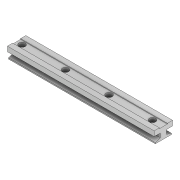
# Autodesk Inventor part: Rail
Saved by Autodesk Inventor 2020 (Build 240168000, 168)
## iProperties
Created: 2020-10-06
Part Number: Rail
Material: Generic
Document SubType Name: Modeling
Designer: ferrerx
Density: 1 g/cm^3
Appearance: Aluminum - Polished
Mass: 26.2987 g
Surface Area: 169.014 cm^2
Volume: 26.2987 cm^3
Author: ferrerx
Autodesk Inventor part; units mm, degrees
ref_plane "YZ Plane" through (0, 0, 0) normal (1, 0, 0) x (0, 1, 0)
ref_plane "XZ Plane" through (0, 0, 0) normal (0, 1, 0) x (-1, 0, 0)
ref_plane "XY Plane" through (0, 0, 0) normal (0, 0, 1) x (1, 0, 0)
sketch "Sketch1" plane through (0, 0, 0) normal (1, 0, 0) x (0, 1, 0)
  line L0 (0, 0) -> (0, -7.42)
  line L1 (0, -7.42) -> (1.0563, -7.42)
  line L2 (1.0563, -7.42) -> (2.51, -2.84)
  line L3 (2.51, -2.84) -> (6.31, -2.84)
  line L4 (6.31, -2.84) -> (6.31, -8.45)
  line L5 (6.31, -8.45) -> (10.81, -8.45)
  line L6 (10.81, -8.45) -> (10.81, -3.65)
  line L7 (10.81, -3.65) -> (10.17, -3.65)
  line L8 (10.17, -3.65) -> (10.17, 0)
  line L9 (0, 0) -> (9.5063, 0) construction
  line L10 (0, 0) -> (0, 7.42)
  line L11 (0, 7.42) -> (1.0563, 7.42)
  line L12 (1.0563, 7.42) -> (2.51, 2.84)
  line L13 (2.51, 2.84) -> (6.31, 2.84)
  line L14 (6.31, 2.84) -> (6.31, 8.45)
  line L15 (6.31, 8.45) -> (10.81, 8.45)
  line L16 (10.81, 8.45) -> (10.81, 3.65)
  line L17 (10.81, 3.65) -> (10.17, 3.65)
  line L18 (10.17, 3.65) -> (10.17, 0)
  dimension "d0" = 8.45
  dimension "d1" = 4.5
  dimension "d2" = 0.64
  dimension "d3" = 3.8
  dimension "d4" = 7.42
  dimension "d5" = 3.65
  dimension "d6" = 10.81
  dimension "d7" = 2.84
  constraints: 38 end point, 8 symmetric about line, 3 perpendicular, 2 parallel, 1 horizontal, 1 vertical
  measures "d0" distance between parallel lines of L9 L5
  measures "d1" distance of L4.end L5.end
  measures "d2" distance of L6.end L7.end
  measures "d3" distance of L2.end L3.end
  measures "d4" distance of L0.start L0.end
  measures "d5" distance of L7.end L8.end
  measures "d6" distance between parallel lines of L0 L6
  measures "d7" distance between parallel lines of L9 L3
extrude "Extrusion1" add sketch "Sketch1" against normal blind 135
sketch "Sketch2" plane through (0, 10.17, 3.65) normal (0, 1, 0) x (1, 0, 0)
  line L0 (0, 3.65) -> (-10, 3.65) construction
  circle A0 centre (-10, 3.65) radius 1.615
  dimension "d10" = 3.23
  dimension "d11" = 10
  constraints: 2 end point, 1 centre point, 1 coincident, 1 horizontal
  measures "d10" diameter of A0
  measures "d11" distance of L0.start L0.end
extrude "Extrusion2" cut sketch "Sketch2" against normal blind 30
sketch "Sketch3" plane through (0, 10.17, 3.65) normal (0, 1, 0) x (1, 0, 0)
  circle A0 centre (-10, 3.65) radius 1.615 projected
  circle A1 centre (-10, 3.65) radius 2.9
  point P0 (0, 3.65)
  dimension "d14" = 5.8
  constraints: 1 centre point, 1 coincident
  measures "d14" diameter of A1
extrude "Extrusion3" cut sketch "Sketch3" against normal blind 3.5
pattern_linear "Rectangular Pattern1" count 8 spacing 40 along (-1, 0, 0) of "Extrusion3", "Extrusion2"
body "Solid1"
